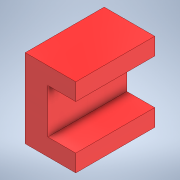
# Autodesk Inventor part: SLIDE
Saved by Autodesk Inventor 2022.4 (Build 264492000, 492)
## iProperties
Created: 2024-01-25
Part Number: SLIDE
Material: Generic
Document SubType Name: Modeling
Designer: t60147996
Density: 1 g/cm^3
Appearance: Light Red
Author: t60147996
Autodesk Inventor part; units mm, degrees
ref_plane "YZ Plane" through (0, 0, 0) normal (1, 0, 0) x (0, 1, 0)
ref_plane "XZ Plane" through (0, 0, 0) normal (0, 1, 0) x (-1, 0, 0)
ref_plane "XY Plane" through (0, 0, 0) normal (0, 0, 1) x (1, 0, 0)
sketch "Sketch1" plane through (0, 0, 0) normal (0, 1, 0) x (-1, 0, 0)
  line L0 (-14.224, 22.225) -> (14.224, 22.225)
  line L1 (14.224, 22.225) -> (14.224, -22.225)
  line L2 (14.224, -22.225) -> (-14.224, -22.225)
  line L3 (-14.224, -22.225) -> (-14.224, 22.225)
  line L4 (-14.224, 22.225) -> (14.224, -22.225) construction
  line L5 (14.224, 22.225) -> (-14.224, -22.225) construction
  point P0 (0, 0)
  dimension "d0" = 28.448
  dimension "d1" = 44.45
  constraints: 12 end point, 2 midpoint, 2 parallel, 1 horizontal, 1 perpendicular
  measures "d0" distance of L1.end L2.end
  measures "d1" distance of L0.end L1.end
extrude "Extrusion1" add sketch "Sketch1" along normal blind 44.45
sketch "Sketch2" plane through (-14.224, 0, 22.225) normal (0, 0, 1) x (1, 0, 0)
  line L0 (12.7, 34.798) -> (53.9197, 34.798)
  line L1 (53.9197, 34.798) -> (53.9197, 9.652)
  line L2 (53.9197, 9.652) -> (12.7, 9.652)
  line L3 (12.7, 9.652) -> (12.7, 34.798)
  line L4 (0, 0) -> (0, 44.45) projected
  line L5 (0, 44.45) -> (28.448, 44.45) projected
  line L6 (0, 0) -> (28.448, 0) projected
  point P0 (14.224, 0)
  dimension "d4" = 12.7
  dimension "d5" = 9.652
  dimension "d6" = 9.652
  constraints: 8 end point, 2 parallel, 1 horizontal, 1 perpendicular
  measures "d4" distance between parallel lines of L3 L4
  measures "d5" distance between parallel lines of L5 L0
  measures "d6" distance between parallel lines of L2 L6
extrude "Extrusion2" cut sketch "Sketch2" against normal blind 44.45
body "Solid1"
